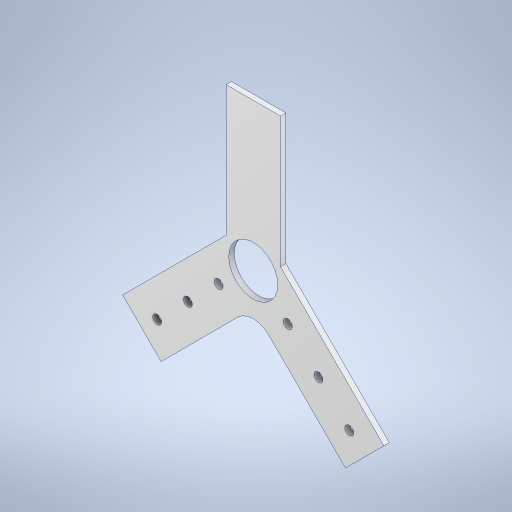
# Autodesk Inventor part: CH-1-HipPivotPlate
Saved by Autodesk Inventor 2023 (Build 270158000, 158)
## iProperties
Created: 2023-03-14
Part Number: CH-1-HipPivotPlate
Material: Aluminum 6061
Document SubType Name: Modeling
Designer: megan
Density: 2.7 g/cm^3
Appearance: Aluminum - Flat
Author: megan
Autodesk Inventor part; units mm, degrees
ref_plane "YZ Plane" through (0, 0, 0) normal (1, 0, 0) x (0, 1, 0)
ref_plane "XZ Plane" through (0, 0, 0) normal (0, 1, 0) x (-1, 0, 0)
ref_plane "XY Plane" through (0, 0, 0) normal (0, 0, 1) x (1, 0, 0)
sketch "Sketch1" plane through (0, 0, 0) normal (0, 0, 1) x (1, 0, 0)
  circle A0 centre (0, 0) radius 14.31
  line L0 (0, -104.7531) -> (0, 117.9978) projected
  line L1 (-53.8815, -72.9315) -> (0, -19.05)
  line L2 (-53.8815, -72.9315) -> (-76.3322, -50.4809)
  line L3 (-76.3322, -50.4809) -> (-15.875, 9.9763)
  line L4 (53.8815, -72.9315) -> (0, -19.05)
  line L5 (53.8815, -72.9315) -> (76.3322, -50.4809)
  line L6 (76.3322, -50.4809) -> (15.875, 9.9763)
  line L7 (-15.875, 9.9763) -> (-15.875, 86.1763)
  line L8 (-15.875, 86.1763) -> (15.875, 86.1763)
  line L9 (15.875, 86.1763) -> (15.875, 9.9763)
  dimension "d0" = 28.62
  dimension "d11" = 76.2
  dimension "d12" = 45
  dimension "d13" = 31.75
  dimension "d28" = 76.2
  dimension "d29" = 15.875
  dimension "d32" = 19.05
  constraints: 18 end point, 2 equal length, 2 parallel, 2 perpendicular, 2 symmetric about line, 1 centre point, 1 coincident, 1 point on line, 1 vertical
  measures "d0" diameter of A0
  measures "d11" distance of L1.start L1.end
  measures "d12" angle of L0 L1
  measures "d13" distance of L1.start L2.end
  measures "d28" distance of L3.end L7.end
  measures "d29" distance between parallel lines of L7 L0
  measures "d32" distance of L1.end point (0, 0)
extrude "Extrusion1" add sketch "Sketch1" along normal blind 3.175 contours A0 L0 L8 L9 L6 L5 L4 | A0 L0 L1 L2 L3 L7 L8
sketch "Sketch2" plane through (0, 0, 3.175) normal (0, 0, 1) x (1, 0, 0)
  line L0 (-76.3322, -50.4809) -> (-53.8815, -72.9315) projected
  line L1 (-65.1069, -61.7062) -> (12.72, 16.1207)
  line L2 (53.8815, -72.9315) -> (76.3322, -50.4809) projected
  line L3 (76.3322, -50.4809) -> (15.875, 9.9763) projected
  line L4 (-15.875, 9.9763) -> (-76.3322, -50.4809) projected
  line L5 (-76.3322, -50.4809) -> (-53.8815, -72.9315) projected
  line L6 (-53.8815, -72.9315) -> (0, -19.05) projected
  line L7 (0, -19.05) -> (53.8815, -72.9315) projected
  circle A0 centre (0, 0) radius 14.31 projected
  circle A1 centre (-56.1266, -52.726) radius 2.65
  circle A2 centre (-38.1661, -34.7654) radius 2.65
  circle A3 centre (-20.2056, -16.8049) radius 2.65
  line L8 (15.875, 9.9763) -> (15.875, 86.1763) projected
  line L9 (15.875, 86.1763) -> (-15.875, 86.1763) projected
  line L10 (-15.875, 86.1763) -> (-15.875, 9.9763) projected
  dimension "d17" = 5.3
  dimension "d18" = 12.7
  dimension "d21" = 25.4
  constraints: 3 centre point, 2 end point, 1 midpoint, 1 perpendicular, 1 point on line, 5 other
  measures "d17" diameter of A1
  measures "d18" distance from line of A1.centre L0
  measures "d21" distance of A1.centre A2.centre
extrude "Extrusion2" cut sketch "Sketch2" against normal blind 3.175 contours A1 L1 | L1 A1 | A2 L1 | L1 A2 | A3 L1 | L1 A3
mirror "Mirror1" about plane through (0, 0, 0) normal (1, 0, 0) of "Extrusion2"
fillet "Fillet1" radius 12.7 1 edges at (0, -19.05, 1.5875)
equation "\"d0\" = bearingDiameter"
equation "\"d28\" = d11"
equation "\"d29\" = 0.5 * d13"
equation "\"d15\" = plateThickness"
equation "\"d17\" = boltDiameter"
equation "\"d26\" = plateThickness"
equation "\"topDiameter\" = 25"
equation "\"shaftLength\" = 76.2"
equation "\"bearingDiameter\" = 28.62"
equation "\"plateThickness\" = 3.175"
equation "\"theta12\" = 100deg"
equation "\"boltDiameter\" = 5.3"
equation "\"gearboxLength\" = 101.6"
equation "\"boltedLength\" = 76.2"
equation "\"innerBoltSpacing\" = 12.7"
equation "\"outerBoltSpacing\" = 12.7"
body "Solid1"
